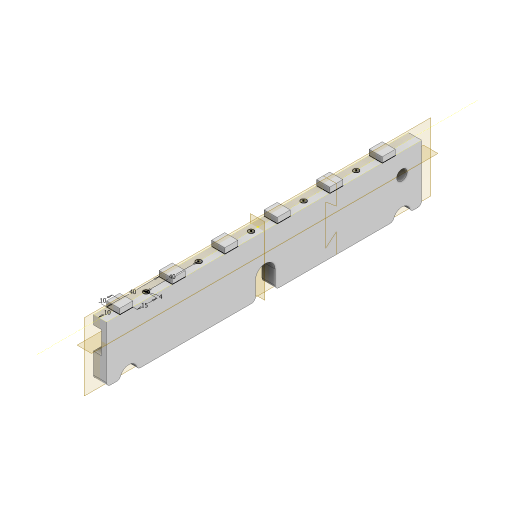
# Autodesk Inventor part: Рельс платформы подъёмника
Saved by Autodesk Inventor 2023.2 (Build 272271030, 271C)
## iProperties
Created: 2025-03-18
Part Number: Рельс платформы подъёмника
Material: Типовые
Document SubType Name: Modeling
Designer: Коноваленко
Density: 1 g/cm^3
Appearance: По умолчанию
Author: Коноваленко
Autodesk Inventor part; units mm, degrees
sketch "Эскиз1" plane through (0, 0, 0) normal (0, 0, 1) x (1, 0, 0)
  line L0 (-5, -14.5) -> (5, -14.5)
  line L1 (5, -14.5) -> (5, 14.5)
  line L2 (-5, -14.5) -> (5, 14.5) construction
  line L3 (5, -14.5) -> (-5, 14.5) construction
  line L4 (-5, 14.5) -> (-5, -14.5)
  line L5 (-5, -7.5) -> (-5, -14.5)
  line L6 (0, 20.3) -> (0, -20.3) construction
  line L7 (5, 14.5) -> (2.5, 14.5)
  line L8 (2.5, 14.5) -> (-5, 14.5)
  point P0 (0, 0)
  dimension "d0" = 10
  dimension "d1" = 29
  constraints: 16 end point, 4 parallel, 2 midpoint, 1 horizontal, 1 perpendicular
  measures "d0" distance of L1.end L3.end
  measures "d1" distance of L0.end L1.end
extrude "Выдавливание1" add sketch "Эскиз1" along normal mid plane 240
sketch "Эскиз2" plane through (-5, 14.5, 120) normal (0, 1, 0) x (1, 0, 0)
  line L0 (0, 240) -> (0, 0) construction
  line L1 (10, 240) -> (10, 0) construction
  line L2 (0, 10) -> (10, 10)
  line L3 (10, 10) -> (10, 20)
  line L4 (10, 20) -> (0, 20)
  line L5 (0, 20) -> (0, 10)
  line L6 (10, 0) -> (0, 0) construction
  line L7 (0, 50) -> (10, 50)
  line L8 (10, 50) -> (10, 60)
  line L9 (10, 60) -> (0, 60)
  line L10 (0, 60) -> (0, 50)
  line L11 (0, 90) -> (10, 90)
  line L12 (10, 90) -> (10, 100)
  line L13 (10, 100) -> (0, 100)
  line L14 (0, 100) -> (0, 90)
  line L15 (0, 130) -> (10, 130)
  line L16 (10, 130) -> (10, 140)
  line L17 (10, 140) -> (0, 140)
  line L18 (0, 140) -> (0, 130)
  line L19 (0, 170) -> (10, 170)
  line L20 (10, 170) -> (10, 180)
  line L21 (10, 180) -> (0, 180)
  line L22 (0, 180) -> (0, 170)
  line L23 (0, 210) -> (10, 210)
  line L24 (10, 210) -> (10, 220)
  line L25 (10, 220) -> (0, 220)
  line L26 (0, 220) -> (0, 210)
  circle A0 centre (5, 35) radius 2
  line L27 (5, 288) -> (5, -48) construction
  circle A1 centre (5, 75) radius 2
  circle A2 centre (5, 115) radius 2
  circle A3 centre (5, 155) radius 2
  circle A4 centre (5, 195) radius 2
  point P0 (5, 120)
  dimension "d13" = 10
  dimension "d14" = 10
  dimension "d17" = 40
  dimension "d24" = 15
  dimension "d25" = 4
  dimension "d28" = 40
  constraints: 48 end point, 5 centre point, 3 point on line, 2 parallel, 2 vertical, 1 horizontal, 1 perpendicular, 48 other
  measures "d13" distance of L2.start L4.end
  measures "d14" distance between parallel lines of L2 L6
  measures "d17" distance of L2.start L7.start
  measures "d24" distance from line of L4 A0.centre
  measures "d25" diameter of A0
  measures "d28" distance of A0.centre A1.centre
extrude "Выдавливание2" add sketch "Эскиз2" along normal blind 4 contours L5 L4 L3 L2 | L10 L9 L8 L7 | L14 L13 L12 L11 | L18 L17 L16 L15 | L22 L21 L20 L19 | L26 L25 L24 L23
sketch "Эскиз3" plane through (-5, -14.5, 120) normal (-1, 0, 0) x (0, 0, 1)
  line L0 (-107.5, 22.1) -> (0, 22.1)
  line L1 (0, 22.1) -> (0, 4.9)
  line L2 (0, 4.9) -> (-107.5, 4.9)
  line L3 (-20, 29) -> (-50, 29) projected
  line L4 (-240, 0) -> (0, 0) projected
  line L5 (0, 29) -> (0, 0) projected
  arc A0 (-107.5, 22.1) -> (-107.5, 4.9) centre (-107.5, 13.5) ccw
  point P0 (-120, 14.5)
  point P1 (-116.1, 13.5)
  point P2 (0, 14.5)
  dimension "d35" = 6.9
  dimension "d36" = 4.9
  constraints: 6 end point, 3 point on circle, 1 centre point, 1 horizontal, 1 midpoint, 1 parallel, 1 perpendicular, 1 point on line, 1 tangent
  measures "d35" distance between parallel lines of L0 L3
  measures "d36" distance between parallel lines of L4 L2
extrude "Выдавливание4" cut sketch "Эскиз3" against normal blind 6
sketch "Эскиз4" plane through (-5, -14.5, -120) normal (-1, 0, 0) x (0, 0, 1)
  circle A0 centre (15, 13.5) radius 4
  line L0 (0, 0) -> (0, 29) projected
  point P0 (120, 14.5)
  dimension "d39" = 8
  dimension "d40" = 15
  constraints: 1 centre point
  measures "d39" diameter of A0
  measures "d40" distance from line of L0 A0.centre
extrude "Выдавливание5" cut sketch "Эскиз4" against normal up to surface (10 mm away)
sketch "Эскиз5" plane through (-5, -14.5, 120) normal (0, -1, 0) x (1, 0, 0)
  line L0 (10, -240) -> (10, 0) projected
  line L1 (0, 0) -> (10, 0) projected
  line L2 (0, -240) -> (0, 0) projected
  line L3 (10, -240) -> (0, -240) projected
  point P0 (5, -120)
extrude "Выдавливание6" add sketch "Эскиз5" along normal blind 14
sketch "Эскиз7" plane through (5, 14.5, -60) normal (1, 0, 0) x (0, 0, -1)
  arc A0 (-156.6892, -43) -> (-169.6892, -43) centre (-163.1892, -43.0184) ccw
  line L0 (60, -43) -> (-180, -43) projected
  circle A1 centre (-163.1892, -43.0184) radius 3 projected
  circle A2 centre (45, -43.0184) radius 3 projected
  arc A3 (51.5, -43) -> (38.5, -43) centre (45, -43.0184) ccw
  line L1 (-66.5946, -43) -> (-51.5946, -43)
  line L2 (-51.5946, -43) -> (-51.5946, -29.2592)
  line L3 (-51.5946, -29.2592) -> (-66.5946, -29.2592) construction
  line L4 (-66.5946, -29.2592) -> (-66.5946, -43)
  circle A4 centre (-59.0946, -29.2592) radius 3 projected
  arc A5 (-51.5946, -29.2592) -> (-66.5946, -29.2592) centre (-59.0946, -29.2592) ccw
  point P0 (-60, -14.5)
  dimension "d58" = 6.5
  dimension "d60" = 6.5
  dimension "d61" = 15
  constraints: 8 end point, 6 point on circle, 5 point on line, 3 centre point, 3 coincident, 2 parallel, 1 horizontal, 1 midpoint, 1 perpendicular
  measures "d58" radius of A0
  measures "d60" radius of A3
  measures "d61" distance of L2.end L3.end
extrude "Выдавливание8" cut sketch "Эскиз7" against normal up to surface (10 mm away) contours L0 A1 A0 | L0 A1 | L0 L4 A5 L2 | L0 A2 A3 | L0 A2 | A4 picked at (-164.103, -42.2994) picked at (44.8799, -41.0887)
fillet "Сопряжение1" radius 3 8 edges at (0, -28.5, -8.4054) (0, -28.5, 6.5946) (0, -28.5, 109.6892) (0, -28.5, 96.6892) (0, -28.5, -98.5) (0, -28.5, -111.5) (0, -28.5, -120) (0, -28.5, 120)
extrude "Выдавливание9" cut sketch "Эскиз2" against normal blind 5.9 contours A0 | A1 | A2
extrude "Выдавливание10" cut sketch "Эскиз2" against normal blind 15 contours A3 | A4
sketch "Эскиз9" plane through (-5, 14.5, 70) normal (-1, 0, 0) x (0, 0, 1)
  line L0 (-90, 0) -> (-120, 0) projected
  line L1 (-125, -11) -> (-117, -4.2872)
  line L2 (-117, -34.7128) -> (-125, -28)
  line L3 (-125, -28) -> (-125, -43)
  line L4 (-165.9923, -43) -> (-81.4054, -43) projected
  line L5 (-81.4054, -43) -> (-165.9923, -43) projected
  line L6 (-117, -4.2872) -> (-117, -34.7128)
  line L7 (-120, 0) -> (-120, 4) projected
  line L8 (-130, 4) -> (-120, 4) projected
  line L9 (-130, 0) -> (-130, 4) projected
  line L10 (-125, -11) -> (-125, 4)
  point P0 (-70, -14.5)
  point P1 (-103, 0)
  dimension "d72" = 50
  dimension "d73" = 15
  dimension "d76" = 8
  dimension "d78" = 50
  dimension "d84" = 5
  dimension "d88" = 50
  dimension "d89" = 15
  constraints: 11 end point, 2 perpendicular, 1 midpoint, 1 point on line
  measures "d72" angle of L2 L3
  measures "d73" distance of L2.end L3.end
  measures "d76" horizontal distance of L2.start L2.end
  measures "d78" angle of L1 L6
  measures "d84" distance between parallel lines of L3 L9
  measures "d88" angle of L1 L10
  measures "d89" distance of L1.start L10.end
surface extrude "ВыдавПврх1" sketch "Эскиз9" against normal up to surface (10 mm away) shown yes curves L3 L2 L6 L1 L10
split body "Разделение3" result two bodies by surface "ВыдавПврх1" first body at (4.5, -14.1667, 54.592)
body "SRF1"
